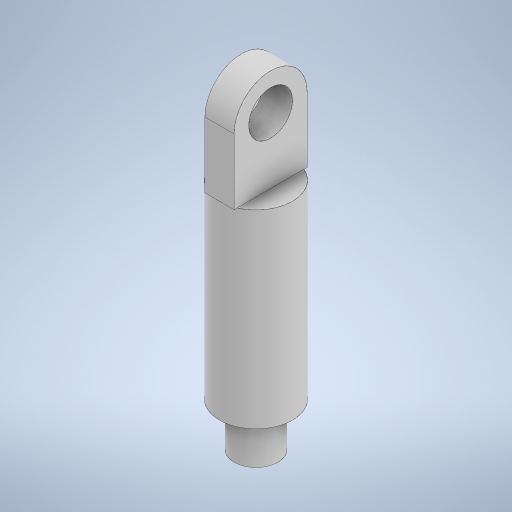
# Autodesk Inventor part: Manipulator Link Type 2
Saved by Autodesk Inventor 2023.2 (Build 272271030, 271C)
## iProperties
Created: 2023-06-26
Part Number: Manipulator Link Type 2
Material: Generic
Document SubType Name: Modeling
Designer: fist5
Density: 1 g/cm^3
Appearance: Default
Author: fist5
Autodesk Inventor part; units mm, degrees
ref_plane "YZ Plane" through (0, 0, 0) normal (1, 0, 0) x (0, 1, 0)
ref_plane "XZ Plane" through (0, 0, 0) normal (0, 1, 0) x (-1, 0, 0)
ref_plane "XY Plane" through (0, 0, 0) normal (0, 0, 1) x (1, 0, 0)
sketch "Sketch7" plane through (0, 0, 0) normal (0, 1, 0) x (-1, 0, 0)
  circle A0 centre (0, 0) radius 25
  circle A1 centre (0, 0) radius 15
  dimension "d19" = 50
  dimension "d20" = 30
  constraints: 2 centre point, 2 coincident
  measures "d19" diameter of A0
  measures "d20" diameter of A1
extrude "Extrusion5" add sketch "Sketch7" against normal blind 30 contours A1
extrude "Extrusion6" add sketch "Sketch7" along normal blind 200 contours A0 | A1
sketch "Sketch8" plane through (0, 0, 0) normal (1, 0, 0) x (0, 1, 0)
  line L0 (200, -25) -> (200, 25) projected
  line L1 (0, -25) -> (0, 25) projected
  line L2 (0, 25) -> (200, 25) projected
  line L3 (0, -25) -> (200, -25) projected
  line L4 (200, -25) -> (200, 25) projected
  line L5 (200, -25) -> (130, -25)
  line L6 (130, -25) -> (130, 25)
  line L7 (130, 25) -> (200, 25)
  line L8 (200, 25) -> (200, -25)
  circle A0 centre (175, 0) radius 25
  circle A1 centre (175, 0) radius 15
  point P0 (0, 0)
  point P1 (0, 0)
  point P2 (175, -25)
  point P3 (175, 25)
  dimension "d25" = 70
  dimension "d26" = 50
  dimension "d27" = 30
  constraints: 8 end point, 2 centre point, 2 parallel, 1 coincident, 1 horizontal, 1 horizontal alignment, 1 midpoint, 1 perpendicular, 1 point on line, 1 tangent
  measures "d25" distance between parallel lines of L6 L0
  measures "d26" diameter of A0
  measures "d27" diameter of A1
extrude "Extrusion7" cut sketch "Sketch8" along normal mid plane 200 contours L3 A0 L0 | A0 L2 L0 | A0 | L3 L6 L2 A0 | A1
extrude "Extrusion8" add sketch "Sketch8" along normal mid plane 20 contours A0 | L3 L6 L2 A0
body "Solid2"
